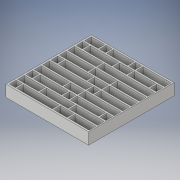
# Autodesk Inventor part: gitter
Saved by Autodesk Inventor 2017 (Build 210142000, 142)
## iProperties
Part Number: gitter
Material: Generisch
Document SubType Name: Modeling
Designer: Primaten
Density: 1 g/cm^3
Appearance: Vorgabe
Author: Primaten
Autodesk Inventor part; units mm, degrees
ref_plane "YZ Plane" through (0, 0, 0) normal (1, 0, 0) x (0, 1, 0)
ref_plane "XZ Plane" through (0, 0, 0) normal (0, 1, 0) x (-1, 0, 0)
ref_plane "XY Plane" through (0, 0, 0) normal (0, 0, 1) x (1, 0, 0)
sketch "Skizze1" plane through (0, 0, 0) normal (0, 0, 1) x (1, 0, 0)
  line L0 (-28.66, 0) -> (171.96, 0) construction
  line L1 (0, -29.6) -> (0, 177.6) construction
  line L2 (3, 3) -> (13.3, 3) construction
  line L3 (13.3, 3) -> (13.3, 14.5) construction
  line L4 (13.3, 14.5) -> (3, 14.5) construction
  line L5 (3, 14.5) -> (3, 3) construction
  line L6 (15.8, 3) -> (26.1, 3) construction
  line L7 (15.8, 14.5) -> (15.8, 3) construction
  line L8 (26.1, 14.5) -> (15.8, 14.5) construction
  line L9 (26.1, 3) -> (26.1, 14.5) construction
  line L10 (28.6, 3) -> (38.9, 3) construction
  line L11 (28.6, 14.5) -> (28.6, 3) construction
  line L12 (38.9, 14.5) -> (28.6, 14.5) construction
  line L13 (38.9, 3) -> (38.9, 14.5) construction
  line L14 (41.4, 3) -> (51.7, 3) construction
  line L15 (41.4, 14.5) -> (41.4, 3) construction
  line L16 (51.7, 14.5) -> (41.4, 14.5) construction
  line L17 (51.7, 3) -> (51.7, 14.5) construction
  line L18 (54.2, 3) -> (64.5, 3) construction
  line L19 (54.2, 14.5) -> (54.2, 3) construction
  line L20 (64.5, 14.5) -> (54.2, 14.5) construction
  line L21 (64.5, 3) -> (64.5, 14.5) construction
  line L22 (67, 3) -> (77.3, 3) construction
  line L23 (67, 14.5) -> (67, 3) construction
  line L24 (77.3, 14.5) -> (67, 14.5) construction
  line L25 (77.3, 3) -> (77.3, 14.5) construction
  line L26 (79.8, 3) -> (90.1, 3) construction
  line L27 (79.8, 14.5) -> (79.8, 3) construction
  line L28 (90.1, 14.5) -> (79.8, 14.5) construction
  line L29 (90.1, 3) -> (90.1, 14.5) construction
  line L30 (92.6, 3) -> (102.9, 3) construction
  line L31 (92.6, 14.5) -> (92.6, 3) construction
  line L32 (102.9, 14.5) -> (92.6, 14.5) construction
  line L33 (102.9, 3) -> (102.9, 14.5) construction
  line L34 (105.4, 3) -> (115.7, 3) construction
  line L35 (105.4, 14.5) -> (105.4, 3) construction
  line L36 (115.7, 14.5) -> (105.4, 14.5) construction
  line L37 (115.7, 3) -> (115.7, 14.5) construction
  line L38 (118.2, 3) -> (128.5, 3) construction
  line L39 (118.2, 14.5) -> (118.2, 3) construction
  line L40 (128.5, 14.5) -> (118.2, 14.5) construction
  line L41 (128.5, 3) -> (128.5, 14.5) construction
  line L42 (131, 3) -> (141.3, 3) construction
  line L43 (131, 14.5) -> (131, 3) construction
  line L44 (141.3, 14.5) -> (131, 14.5) construction
  line L45 (141.3, 3) -> (141.3, 14.5) construction
  line L46 (3, 17.5) -> (13.3, 17.5) construction
  line L47 (3, 29) -> (3, 17.5) construction
  line L48 (13.3, 29) -> (3, 29) construction
  line L49 (13.3, 17.5) -> (13.3, 29) construction
  line L50 (15.8, 17.5) -> (26.1, 17.5) construction
  line L51 (15.8, 29) -> (15.8, 17.5) construction
  line L52 (26.1, 29) -> (15.8, 29) construction
  line L53 (26.1, 17.5) -> (26.1, 29) construction
  line L54 (28.6, 17.5) -> (38.9, 17.5) construction
  line L55 (28.6, 29) -> (28.6, 17.5) construction
  line L56 (38.9, 29) -> (28.6, 29) construction
  line L57 (38.9, 17.5) -> (38.9, 29) construction
  line L58 (41.4, 17.5) -> (51.7, 17.5) construction
  line L59 (41.4, 29) -> (41.4, 17.5) construction
  line L60 (51.7, 29) -> (41.4, 29) construction
  line L61 (51.7, 17.5) -> (51.7, 29) construction
  line L62 (54.2, 17.5) -> (64.5, 17.5) construction
  line L63 (54.2, 29) -> (54.2, 17.5) construction
  line L64 (64.5, 29) -> (54.2, 29) construction
  line L65 (64.5, 17.5) -> (64.5, 29) construction
  line L66 (67, 17.5) -> (77.3, 17.5) construction
  line L67 (67, 29) -> (67, 17.5) construction
  line L68 (77.3, 29) -> (67, 29) construction
  line L69 (77.3, 17.5) -> (77.3, 29) construction
  line L70 (79.8, 17.5) -> (90.1, 17.5) construction
  line L71 (79.8, 29) -> (79.8, 17.5) construction
  line L72 (90.1, 29) -> (79.8, 29) construction
  line L73 (90.1, 17.5) -> (90.1, 29) construction
  line L74 (92.6, 17.5) -> (102.9, 17.5) construction
  line L75 (92.6, 29) -> (92.6, 17.5) construction
  line L76 (102.9, 29) -> (92.6, 29) construction
  line L77 (102.9, 17.5) -> (102.9, 29) construction
  line L78 (105.4, 17.5) -> (115.7, 17.5) construction
  line L79 (105.4, 29) -> (105.4, 17.5) construction
  line L80 (115.7, 29) -> (105.4, 29) construction
  line L81 (115.7, 17.5) -> (115.7, 29) construction
  line L82 (118.2, 17.5) -> (128.5, 17.5) construction
  line L83 (118.2, 29) -> (118.2, 17.5) construction
  line L84 (128.5, 29) -> (118.2, 29) construction
  line L85 (128.5, 17.5) -> (128.5, 29) construction
  line L86 (131, 17.5) -> (141.3, 17.5) construction
  line L87 (131, 29) -> (131, 17.5) construction
  line L88 (141.3, 29) -> (131, 29) construction
  line L89 (141.3, 17.5) -> (141.3, 29) construction
  line L90 (3, 32) -> (13.3, 32) construction
  line L91 (3, 43.5) -> (3, 32) construction
  line L92 (13.3, 43.5) -> (3, 43.5) construction
  line L93 (13.3, 32) -> (13.3, 43.5) construction
  line L94 (15.8, 32) -> (26.1, 32) construction
  line L95 (15.8, 43.5) -> (15.8, 32) construction
  line L96 (26.1, 43.5) -> (15.8, 43.5) construction
  line L97 (26.1, 32) -> (26.1, 43.5) construction
  line L98 (28.6, 32) -> (38.9, 32) construction
  line L99 (28.6, 43.5) -> (28.6, 32) construction
  line L100 (38.9, 43.5) -> (28.6, 43.5) construction
  line L101 (38.9, 32) -> (38.9, 43.5) construction
  line L102 (41.4, 32) -> (51.7, 32) construction
  line L103 (41.4, 43.5) -> (41.4, 32) construction
  line L104 (51.7, 43.5) -> (41.4, 43.5) construction
  line L105 (51.7, 32) -> (51.7, 43.5) construction
  line L106 (54.2, 32) -> (64.5, 32) construction
  line L107 (54.2, 43.5) -> (54.2, 32) construction
  line L108 (64.5, 43.5) -> (54.2, 43.5) construction
  line L109 (64.5, 32) -> (64.5, 43.5) construction
  line L110 (67, 32) -> (77.3, 32) construction
  line L111 (67, 43.5) -> (67, 32) construction
  line L112 (77.3, 43.5) -> (67, 43.5) construction
  line L113 (77.3, 32) -> (77.3, 43.5) construction
  line L114 (79.8, 32) -> (90.1, 32) construction
  line L115 (79.8, 43.5) -> (79.8, 32) construction
  line L116 (90.1, 43.5) -> (79.8, 43.5) construction
  line L117 (90.1, 32) -> (90.1, 43.5) construction
  line L118 (92.6, 32) -> (102.9, 32) construction
  line L119 (92.6, 43.5) -> (92.6, 32) construction
  line L120 (102.9, 43.5) -> (92.6, 43.5) construction
  line L121 (102.9, 32) -> (102.9, 43.5) construction
  line L122 (105.4, 32) -> (115.7, 32) construction
  line L123 (105.4, 43.5) -> (105.4, 32) construction
  line L124 (115.7, 43.5) -> (105.4, 43.5) construction
  line L125 (115.7, 32) -> (115.7, 43.5) construction
  line L126 (118.2, 32) -> (128.5, 32) construction
  line L127 (118.2, 43.5) -> (118.2, 32) construction
  line L128 (128.5, 43.5) -> (118.2, 43.5) construction
  line L129 (128.5, 32) -> (128.5, 43.5) construction
  line L130 (131, 32) -> (141.3, 32) construction
  line L131 (131, 43.5) -> (131, 32) construction
  line L132 (141.3, 43.5) -> (131, 43.5) construction
  line L133 (141.3, 32) -> (141.3, 43.5) construction
  line L134 (3, 46.5) -> (13.3, 46.5) construction
  line L135 (3, 58) -> (3, 46.5) construction
  line L136 (13.3, 58) -> (3, 58) construction
  line L137 (13.3, 46.5) -> (13.3, 58) construction
  line L138 (15.8, 46.5) -> (26.1, 46.5) construction
  line L139 (15.8, 58) -> (15.8, 46.5) construction
  line L140 (26.1, 58) -> (15.8, 58) construction
  line L141 (26.1, 46.5) -> (26.1, 58) construction
  line L142 (28.6, 46.5) -> (38.9, 46.5) construction
  line L143 (28.6, 58) -> (28.6, 46.5) construction
  line L144 (38.9, 58) -> (28.6, 58) construction
  line L145 (38.9, 46.5) -> (38.9, 58) construction
  line L146 (41.4, 46.5) -> (51.7, 46.5) construction
  line L147 (41.4, 58) -> (41.4, 46.5) construction
  line L148 (51.7, 58) -> (41.4, 58) construction
  line L149 (51.7, 46.5) -> (51.7, 58) construction
  line L150 (54.2, 46.5) -> (64.5, 46.5) construction
  line L151 (54.2, 58) -> (54.2, 46.5) construction
  line L152 (64.5, 58) -> (54.2, 58) construction
  line L153 (64.5, 46.5) -> (64.5, 58) construction
  line L154 (67, 46.5) -> (77.3, 46.5) construction
  line L155 (67, 58) -> (67, 46.5) construction
  line L156 (77.3, 58) -> (67, 58) construction
  line L157 (77.3, 46.5) -> (77.3, 58) construction
  line L158 (79.8, 46.5) -> (90.1, 46.5) construction
  line L159 (79.8, 58) -> (79.8, 46.5) construction
  line L160 (90.1, 58) -> (79.8, 58) construction
  line L161 (90.1, 46.5) -> (90.1, 58) construction
  line L162 (92.6, 46.5) -> (102.9, 46.5) construction
  line L163 (92.6, 58) -> (92.6, 46.5) construction
  line L164 (102.9, 58) -> (92.6, 58) construction
  line L165 (102.9, 46.5) -> (102.9, 58) construction
  line L166 (105.4, 46.5) -> (115.7, 46.5) construction
  line L167 (105.4, 58) -> (105.4, 46.5) construction
  line L168 (115.7, 58) -> (105.4, 58) construction
  line L169 (115.7, 46.5) -> (115.7, 58) construction
  line L170 (118.2, 46.5) -> (128.5, 46.5) construction
  line L171 (118.2, 58) -> (118.2, 46.5) construction
  line L172 (128.5, 58) -> (118.2, 58) construction
  line L173 (128.5, 46.5) -> (128.5, 58) construction
  line L174 (131, 46.5) -> (141.3, 46.5) construction
  line L175 (131, 58) -> (131, 46.5) construction
  line L176 (141.3, 58) -> (131, 58) construction
  line L177 (141.3, 46.5) -> (141.3, 58) construction
  line L178 (3, 61) -> (13.3, 61) construction
  line L179 (3, 72.5) -> (3, 61) construction
  line L180 (13.3, 72.5) -> (3, 72.5) construction
  line L181 (13.3, 61) -> (13.3, 72.5) construction
  line L182 (15.8, 61) -> (26.1, 61) construction
  line L183 (15.8, 72.5) -> (15.8, 61) construction
  line L184 (26.1, 72.5) -> (15.8, 72.5) construction
  line L185 (26.1, 61) -> (26.1, 72.5) construction
  line L186 (28.6, 61) -> (38.9, 61) construction
  line L187 (28.6, 72.5) -> (28.6, 61) construction
  line L188 (38.9, 72.5) -> (28.6, 72.5) construction
  line L189 (38.9, 61) -> (38.9, 72.5) construction
  line L190 (41.4, 61) -> (51.7, 61) construction
  line L191 (41.4, 72.5) -> (41.4, 61) construction
  line L192 (51.7, 72.5) -> (41.4, 72.5) construction
  line L193 (51.7, 61) -> (51.7, 72.5) construction
  line L194 (54.2, 61) -> (64.5, 61) construction
  line L195 (54.2, 72.5) -> (54.2, 61) construction
  line L196 (64.5, 72.5) -> (54.2, 72.5) construction
  line L197 (64.5, 61) -> (64.5, 72.5) construction
  line L198 (67, 61) -> (77.3, 61) construction
  line L199 (67, 72.5) -> (67, 61) construction
  line L200 (77.3, 72.5) -> (67, 72.5) construction
  line L201 (77.3, 61) -> (77.3, 72.5) construction
  line L202 (79.8, 61) -> (90.1, 61) construction
  line L203 (79.8, 72.5) -> (79.8, 61) construction
  line L204 (90.1, 72.5) -> (79.8, 72.5) construction
  line L205 (90.1, 61) -> (90.1, 72.5) construction
  line L206 (92.6, 61) -> (102.9, 61) construction
  line L207 (92.6, 72.5) -> (92.6, 61) construction
  line L208 (102.9, 72.5) -> (92.6, 72.5) construction
  line L209 (102.9, 61) -> (102.9, 72.5) construction
  line L210 (105.4, 61) -> (115.7, 61) construction
  line L211 (105.4, 72.5) -> (105.4, 61) construction
  line L212 (115.7, 72.5) -> (105.4, 72.5) construction
  line L213 (115.7, 61) -> (115.7, 72.5) construction
  line L214 (118.2, 61) -> (128.5, 61) construction
  line L215 (118.2, 72.5) -> (118.2, 61) construction
  line L216 (128.5, 72.5) -> (118.2, 72.5) construction
  line L217 (128.5, 61) -> (128.5, 72.5) construction
  line L218 (131, 61) -> (141.3, 61) construction
  line L219 (131, 72.5) -> (131, 61) construction
  line L220 (141.3, 72.5) -> (131, 72.5) construction
  line L221 (141.3, 61) -> (141.3, 72.5) construction
  line L222 (3, 75.5) -> (13.3, 75.5) construction
  line L223 (3, 87) -> (3, 75.5) construction
  line L224 (13.3, 87) -> (3, 87) construction
  line L225 (13.3, 75.5) -> (13.3, 87) construction
  line L226 (15.8, 75.5) -> (26.1, 75.5) construction
  line L227 (15.8, 87) -> (15.8, 75.5) construction
  line L228 (26.1, 87) -> (15.8, 87) construction
  line L229 (26.1, 75.5) -> (26.1, 87) construction
  line L230 (28.6, 75.5) -> (38.9, 75.5) construction
  line L231 (28.6, 87) -> (28.6, 75.5) construction
  line L232 (38.9, 87) -> (28.6, 87) construction
  line L233 (38.9, 75.5) -> (38.9, 87) construction
  line L234 (41.4, 75.5) -> (51.7, 75.5) construction
  line L235 (41.4, 87) -> (41.4, 75.5) construction
  line L236 (51.7, 87) -> (41.4, 87) construction
  line L237 (51.7, 75.5) -> (51.7, 87) construction
  line L238 (54.2, 75.5) -> (64.5, 75.5) construction
  line L239 (54.2, 87) -> (54.2, 75.5) construction
  line L240 (64.5, 87) -> (54.2, 87) construction
  line L241 (64.5, 75.5) -> (64.5, 87) construction
  line L242 (67, 75.5) -> (77.3, 75.5) construction
  line L243 (67, 87) -> (67, 75.5) construction
  line L244 (77.3, 87) -> (67, 87) construction
  line L245 (77.3, 75.5) -> (77.3, 87) construction
  line L246 (79.8, 75.5) -> (90.1, 75.5) construction
  line L247 (79.8, 87) -> (79.8, 75.5) construction
  line L248 (90.1, 87) -> (79.8, 87) construction
  line L249 (90.1, 75.5) -> (90.1, 87) construction
  line L250 (92.6, 75.5) -> (102.9, 75.5) construction
  line L251 (92.6, 87) -> (92.6, 75.5) construction
  line L252 (102.9, 87) -> (92.6, 87) construction
  line L253 (102.9, 75.5) -> (102.9, 87) construction
  line L254 (105.4, 75.5) -> (115.7, 75.5) construction
  line L255 (105.4, 87) -> (105.4, 75.5) construction
  line L256 (115.7, 87) -> (105.4, 87) construction
  line L257 (115.7, 75.5) -> (115.7, 87) construction
  line L258 (118.2, 75.5) -> (128.5, 75.5) construction
  line L259 (118.2, 87) -> (118.2, 75.5) construction
  line L260 (128.5, 87) -> (118.2, 87) construction
  line L261 (128.5, 75.5) -> (128.5, 87) construction
  line L262 (131, 75.5) -> (141.3, 75.5) construction
  line L263 (131, 87) -> (131, 75.5) construction
  line L264 (141.3, 87) -> (131, 87) construction
  line L265 (141.3, 75.5) -> (141.3, 87) construction
  line L266 (3, 90) -> (13.3, 90) construction
  line L267 (3, 101.5) -> (3, 90) construction
  line L268 (13.3, 101.5) -> (3, 101.5) construction
  line L269 (13.3, 90) -> (13.3, 101.5) construction
  line L270 (15.8, 90) -> (26.1, 90) construction
  line L271 (15.8, 101.5) -> (15.8, 90) construction
  line L272 (26.1, 101.5) -> (15.8, 101.5) construction
  line L273 (26.1, 90) -> (26.1, 101.5) construction
  line L274 (28.6, 90) -> (38.9, 90) construction
  line L275 (28.6, 101.5) -> (28.6, 90) construction
  line L276 (38.9, 101.5) -> (28.6, 101.5) construction
  line L277 (38.9, 90) -> (38.9, 101.5) construction
  line L278 (41.4, 90) -> (51.7, 90) construction
  line L279 (41.4, 101.5) -> (41.4, 90) construction
  line L280 (51.7, 101.5) -> (41.4, 101.5) construction
  line L281 (51.7, 90) -> (51.7, 101.5) construction
  line L282 (54.2, 90) -> (64.5, 90) construction
  line L283 (54.2, 101.5) -> (54.2, 90) construction
  line L284 (64.5, 101.5) -> (54.2, 101.5) construction
  line L285 (64.5, 90) -> (64.5, 101.5) construction
  line L286 (67, 90) -> (77.3, 90) construction
  line L287 (67, 101.5) -> (67, 90) construction
  line L288 (77.3, 101.5) -> (67, 101.5) construction
  line L289 (77.3, 90) -> (77.3, 101.5) construction
  line L290 (79.8, 90) -> (90.1, 90) construction
  line L291 (79.8, 101.5) -> (79.8, 90) construction
  line L292 (90.1, 101.5) -> (79.8, 101.5) construction
  line L293 (90.1, 90) -> (90.1, 101.5) construction
  line L294 (92.6, 90) -> (102.9, 90) construction
  line L295 (92.6, 101.5) -> (92.6, 90) construction
  line L296 (102.9, 101.5) -> (92.6, 101.5) construction
  line L297 (102.9, 90) -> (102.9, 101.5) construction
  line L298 (105.4, 90) -> (115.7, 90) construction
  line L299 (105.4, 101.5) -> (105.4, 90) construction
  line L300 (115.7, 101.5) -> (105.4, 101.5) construction
  line L301 (115.7, 90) -> (115.7, 101.5) construction
  line L302 (118.2, 90) -> (128.5, 90) construction
  line L303 (118.2, 101.5) -> (118.2, 90) construction
  line L304 (128.5, 101.5) -> (118.2, 101.5) construction
  line L305 (128.5, 90) -> (128.5, 101.5) construction
  line L306 (131, 90) -> (141.3, 90) construction
  line L307 (131, 101.5) -> (131, 90) construction
  line L308 (141.3, 101.5) -> (131, 101.5) construction
  line L309 (141.3, 90) -> (141.3, 101.5) construction
  line L310 (3, 104.5) -> (13.3, 104.5) construction
  line L311 (3, 116) -> (3, 104.5) construction
  line L312 (13.3, 116) -> (3, 116) construction
  line L313 (13.3, 104.5) -> (13.3, 116) construction
  line L314 (15.8, 104.5) -> (26.1, 104.5) construction
  line L315 (15.8, 116) -> (15.8, 104.5) construction
  line L316 (26.1, 116) -> (15.8, 116) construction
  line L317 (26.1, 104.5) -> (26.1, 116) construction
  line L318 (28.6, 104.5) -> (38.9, 104.5) construction
  line L319 (28.6, 116) -> (28.6, 104.5) construction
  line L320 (38.9, 116) -> (28.6, 116) construction
  line L321 (38.9, 104.5) -> (38.9, 116) construction
  line L322 (41.4, 104.5) -> (51.7, 104.5) construction
  line L323 (41.4, 116) -> (41.4, 104.5) construction
  line L324 (51.7, 116) -> (41.4, 116) construction
  line L325 (51.7, 104.5) -> (51.7, 116) construction
  line L326 (54.2, 104.5) -> (64.5, 104.5) construction
  line L327 (54.2, 116) -> (54.2, 104.5) construction
  line L328 (64.5, 116) -> (54.2, 116) construction
  line L329 (64.5, 104.5) -> (64.5, 116) construction
  line L330 (67, 104.5) -> (77.3, 104.5) construction
  line L331 (67, 116) -> (67, 104.5) construction
  line L332 (77.3, 116) -> (67, 116) construction
  line L333 (77.3, 104.5) -> (77.3, 116) construction
  line L334 (79.8, 104.5) -> (90.1, 104.5) construction
  line L335 (79.8, 116) -> (79.8, 104.5) construction
  line L336 (90.1, 116) -> (79.8, 116) construction
  line L337 (90.1, 104.5) -> (90.1, 116) construction
  line L338 (92.6, 104.5) -> (102.9, 104.5) construction
  line L339 (92.6, 116) -> (92.6, 104.5) construction
  line L340 (102.9, 116) -> (92.6, 116) construction
  line L341 (102.9, 104.5) -> (102.9, 116) construction
  line L342 (105.4, 104.5) -> (115.7, 104.5) construction
  line L343 (105.4, 116) -> (105.4, 104.5) construction
  line L344 (115.7, 116) -> (105.4, 116) construction
  line L345 (115.7, 104.5) -> (115.7, 116) construction
  line L346 (118.2, 104.5) -> (128.5, 104.5) construction
  line L347 (118.2, 116) -> (118.2, 104.5) construction
  line L348 (128.5, 116) -> (118.2, 116) construction
  line L349 (128.5, 104.5) -> (128.5, 116) construction
  line L350 (131, 104.5) -> (141.3, 104.5) construction
  line L351 (131, 116) -> (131, 104.5) construction
  line L352 (141.3, 116) -> (131, 116) construction
  line L353 (141.3, 104.5) -> (141.3, 116) construction
  line L354 (3, 119) -> (13.3, 119) construction
  line L355 (3, 130.5) -> (3, 119) construction
  line L356 (13.3, 130.5) -> (3, 130.5) construction
  line L357 (13.3, 119) -> (13.3, 130.5) construction
  line L358 (15.8, 119) -> (26.1, 119) construction
  line L359 (15.8, 130.5) -> (15.8, 119) construction
  line L360 (26.1, 130.5) -> (15.8, 130.5) construction
  line L361 (26.1, 119) -> (26.1, 130.5) construction
  line L362 (28.6, 119) -> (38.9, 119) construction
  line L363 (28.6, 130.5) -> (28.6, 119) construction
  line L364 (38.9, 130.5) -> (28.6, 130.5) construction
  line L365 (38.9, 119) -> (38.9, 130.5) construction
  line L366 (41.4, 119) -> (51.7, 119) construction
  line L367 (41.4, 130.5) -> (41.4, 119) construction
  line L368 (51.7, 130.5) -> (41.4, 130.5) construction
  line L369 (51.7, 119) -> (51.7, 130.5) construction
  line L370 (54.2, 119) -> (64.5, 119) construction
  line L371 (54.2, 130.5) -> (54.2, 119) construction
  line L372 (64.5, 130.5) -> (54.2, 130.5) construction
  line L373 (64.5, 119) -> (64.5, 130.5) construction
  line L374 (67, 119) -> (77.3, 119) construction
  line L375 (67, 130.5) -> (67, 119) construction
  line L376 (77.3, 130.5) -> (67, 130.5) construction
  line L377 (77.3, 119) -> (77.3, 130.5) construction
  line L378 (79.8, 119) -> (90.1, 119) construction
  line L379 (79.8, 130.5) -> (79.8, 119) construction
  line L380 (90.1, 130.5) -> (79.8, 130.5) construction
  line L381 (90.1, 119) -> (90.1, 130.5) construction
  line L382 (92.6, 119) -> (102.9, 119) construction
  line L383 (92.6, 130.5) -> (92.6, 119) construction
  line L384 (102.9, 130.5) -> (92.6, 130.5) construction
  line L385 (102.9, 119) -> (102.9, 130.5) construction
  line L386 (105.4, 119) -> (115.7, 119) construction
  line L387 (105.4, 130.5) -> (105.4, 119) construction
  line L388 (115.7, 130.5) -> (105.4, 130.5) construction
  line L389 (115.7, 119) -> (115.7, 130.5) construction
  line L390 (118.2, 119) -> (128.5, 119) construction
  line L391 (118.2, 130.5) -> (118.2, 119) construction
  line L392 (128.5, 130.5) -> (118.2, 130.5) construction
  line L393 (128.5, 119) -> (128.5, 130.5) construction
  line L394 (131, 119) -> (141.3, 119) construction
  line L395 (131, 130.5) -> (131, 119) construction
  line L396 (141.3, 130.5) -> (131, 130.5) construction
  line L397 (141.3, 119) -> (141.3, 130.5) construction
  line L398 (3, 133.5) -> (13.3, 133.5) construction
  line L399 (3, 145) -> (3, 133.5) construction
  line L400 (13.3, 145) -> (3, 145) construction
  line L401 (13.3, 133.5) -> (13.3, 145) construction
  line L402 (15.8, 133.5) -> (26.1, 133.5) construction
  line L403 (15.8, 145) -> (15.8, 133.5) construction
  line L404 (26.1, 145) -> (15.8, 145) construction
  line L405 (26.1, 133.5) -> (26.1, 145) construction
  line L406 (28.6, 133.5) -> (38.9, 133.5) construction
  line L407 (28.6, 145) -> (28.6, 133.5) construction
  line L408 (38.9, 145) -> (28.6, 145) construction
  line L409 (38.9, 133.5) -> (38.9, 145) construction
  line L410 (41.4, 133.5) -> (51.7, 133.5) construction
  line L411 (41.4, 145) -> (41.4, 133.5) construction
  line L412 (51.7, 145) -> (41.4, 145) construction
  line L413 (51.7, 133.5) -> (51.7, 145) construction
  line L414 (54.2, 133.5) -> (64.5, 133.5) construction
  line L415 (54.2, 145) -> (54.2, 133.5) construction
  line L416 (64.5, 145) -> (54.2, 145) construction
  line L417 (64.5, 133.5) -> (64.5, 145) construction
  line L418 (67, 133.5) -> (77.3, 133.5) construction
  line L419 (67, 145) -> (67, 133.5) construction
  line L420 (77.3, 145) -> (67, 145) construction
  line L421 (77.3, 133.5) -> (77.3, 145) construction
  line L422 (79.8, 133.5) -> (90.1, 133.5) construction
  line L423 (79.8, 145) -> (79.8, 133.5) construction
  line L424 (90.1, 145) -> (79.8, 145) construction
  line L425 (90.1, 133.5) -> (90.1, 145) construction
  line L426 (92.6, 133.5) -> (102.9, 133.5) construction
  line L427 (92.6, 145) -> (92.6, 133.5) construction
  line L428 (102.9, 145) -> (92.6, 145) construction
  line L429 (102.9, 133.5) -> (102.9, 145) construction
  line L430 (105.4, 133.5) -> (115.7, 133.5) construction
  line L431 (105.4, 145) -> (105.4, 133.5) construction
  line L432 (115.7, 145) -> (105.4, 145) construction
  line L433 (115.7, 133.5) -> (115.7, 145) construction
  line L434 (118.2, 133.5) -> (128.5, 133.5) construction
  line L435 (118.2, 145) -> (118.2, 133.5) construction
  line L436 (128.5, 145) -> (118.2, 145) construction
  line L437 (128.5, 133.5) -> (128.5, 145) construction
  line L438 (131, 133.5) -> (141.3, 133.5) construction
  line L439 (131, 145) -> (131, 133.5) construction
  line L440 (141.3, 145) -> (131, 145) construction
  line L441 (141.3, 133.5) -> (141.3, 145) construction
  line L442 (0, 0) -> (143.3, 0) construction
  line L443 (143.3, 0) -> (143.3, 148) construction
  line L444 (143.3, 148) -> (0, 148) construction
  line L445 (0, 148) -> (0, 0) construction
  line L446 (0, 0) -> (143.3, 0)
  line L447 (143.3, 0) -> (143.3, 148)
  line L448 (143.3, 148) -> (0, 148)
  line L449 (0, 148) -> (0, 0)
  line L450 (3, 145) -> (26.1, 145)
  line L451 (26.1, 145) -> (26.1, 133.5)
  line L452 (26.1, 133.5) -> (3, 133.5)
  line L453 (3, 133.5) -> (3, 145)
  line L454 (28.6, 145) -> (38.9, 145)
  line L455 (38.9, 145) -> (38.9, 133.5)
  line L456 (38.9, 133.5) -> (28.6, 133.5)
  line L457 (28.6, 133.5) -> (28.6, 145)
  line L458 (41.4, 145) -> (77.3, 145)
  line L459 (77.3, 145) -> (77.3, 133.5)
  line L460 (77.3, 133.5) -> (41.4, 133.5)
  line L461 (41.4, 133.5) -> (41.4, 145)
  line L462 (79.8, 145) -> (90.1, 145)
  line L463 (90.1, 145) -> (90.1, 133.5)
  line L464 (90.1, 133.5) -> (79.8, 133.5)
  line L465 (79.8, 133.5) -> (79.8, 145)
  line L466 (90.1, 130.5) -> (67, 130.5)
  line L467 (67, 130.5) -> (67, 119)
  line L468 (67, 119) -> (90.1, 119)
  line L469 (90.1, 119) -> (90.1, 130.5)
  line L470 (92.6, 133.5) -> (141.3, 133.5)
  line L471 (141.3, 133.5) -> (141.3, 145)
  line L472 (141.3, 145) -> (92.6, 145)
  line L473 (92.6, 145) -> (92.6, 133.5)
  line L474 (131, 130.5) -> (141.3, 130.5)
  line L475 (141.3, 130.5) -> (141.3, 119)
  line L476 (141.3, 119) -> (131, 119)
  line L477 (131, 119) -> (131, 130.5)
  line L478 (128.5, 130.5) -> (92.6, 130.5)
  line L479 (92.6, 130.5) -> (92.6, 119)
  line L480 (92.6, 119) -> (128.5, 119)
  line L481 (128.5, 119) -> (128.5, 130.5)
  line L482 (51.7, 116) -> (3, 116)
  line L483 (3, 116) -> (3, 104.5)
  line L484 (3, 104.5) -> (51.7, 104.5)
  line L485 (51.7, 104.5) -> (51.7, 116)
  line L486 (54.2, 116) -> (141.3, 116)
  line L487 (141.3, 116) -> (141.3, 104.5)
  line L488 (141.3, 104.5) -> (54.2, 104.5)
  line L489 (54.2, 104.5) -> (54.2, 116)
  line L490 (13.3, 130.5) -> (3, 130.5)
  line L491 (3, 130.5) -> (3, 119)
  line L492 (3, 119) -> (13.3, 119)
  line L493 (13.3, 119) -> (13.3, 130.5)
  line L494 (15.8, 119) -> (64.5, 119)
  line L495 (64.5, 119) -> (64.5, 130.5)
  line L496 (64.5, 130.5) -> (15.8, 130.5)
  line L497 (15.8, 130.5) -> (15.8, 119)
  line L498 (51.7, 101.5) -> (3, 101.5)
  line L499 (3, 101.5) -> (3, 90)
  line L500 (3, 90) -> (51.7, 90)
  line L501 (51.7, 90) -> (51.7, 101.5)
  line L502 (54.2, 101.5) -> (90.1, 101.5)
  line L503 (90.1, 101.5) -> (90.1, 90)
  line L504 (90.1, 90) -> (54.2, 90)
  line L505 (54.2, 90) -> (54.2, 101.5)
  line L506 (92.6, 101.5) -> (141.3, 101.5)
  line L507 (141.3, 101.5) -> (141.3, 90)
  line L508 (141.3, 90) -> (92.6, 90)
  line L509 (92.6, 90) -> (92.6, 101.5)
  line L510 (3, 87) -> (13.3, 87)
  line L511 (13.3, 87) -> (13.3, 75.5)
  line L512 (13.3, 75.5) -> (3, 75.5)
  line L513 (3, 75.5) -> (3, 87)
  line L514 (15.8, 87) -> (64.5, 87)
  line L515 (64.5, 87) -> (64.5, 75.5)
  line L516 (64.5, 75.5) -> (15.8, 75.5)
  line L517 (15.8, 75.5) -> (15.8, 87)
  line L518 (67, 87) -> (90.1, 87)
  line L519 (90.1, 87) -> (90.1, 75.5)
  line L520 (90.1, 75.5) -> (67, 75.5)
  line L521 (67, 75.5) -> (67, 87)
  line L522 (92.6, 87) -> (141.3, 87)
  line L523 (141.3, 87) -> (141.3, 75.5)
  line L524 (141.3, 75.5) -> (92.6, 75.5)
  line L525 (92.6, 75.5) -> (92.6, 87)
  line L526 (79.8, 72.5) -> (90.1, 72.5)
  line L527 (90.1, 72.5) -> (90.1, 61)
  line L528 (90.1, 61) -> (79.8, 61)
  line L529 (79.8, 61) -> (79.8, 72.5)
  line L530 (92.6, 61) -> (141.3, 61)
  line L531 (141.3, 61) -> (141.3, 72.5)
  line L532 (141.3, 72.5) -> (92.6, 72.5)
  line L533 (92.6, 72.5) -> (92.6, 61)
  line L534 (77.3, 72.5) -> (3, 72.5)
  line L535 (3, 72.5) -> (3, 61)
  line L536 (3, 61) -> (77.3, 61)
  line L537 (77.3, 61) -> (77.3, 72.5)
  line L538 (3, 58) -> (51.7, 58)
  line L539 (51.7, 58) -> (51.7, 46.5)
  line L540 (51.7, 46.5) -> (3, 46.5)
  line L541 (3, 46.5) -> (3, 58)
  line L542 (54.2, 58) -> (77.3, 58)
  line L543 (77.3, 58) -> (77.3, 46.5)
  line L544 (77.3, 46.5) -> (54.2, 46.5)
  line L545 (54.2, 46.5) -> (54.2, 58)
  line L546 (79.8, 58) -> (141.3, 58)
  line L547 (141.3, 58) -> (141.3, 46.5)
  line L548 (141.3, 46.5) -> (79.8, 46.5)
  line L549 (79.8, 46.5) -> (79.8, 58)
  line L550 (77.3, 43.5) -> (67, 43.5)
  line L551 (67, 43.5) -> (67, 32)
  line L552 (67, 32) -> (77.3, 32)
  line L553 (77.3, 32) -> (77.3, 43.5)
  line L554 (64.5, 43.5) -> (15.8, 43.5)
  line L555 (15.8, 43.5) -> (15.8, 32)
  line L556 (15.8, 32) -> (64.5, 32)
  line L557 (64.5, 32) -> (64.5, 43.5)
  line L558 (13.3, 43.5) -> (3, 43.5)
  line L559 (3, 43.5) -> (3, 32)
  line L560 (3, 32) -> (13.3, 32)
  line L561 (13.3, 32) -> (13.3, 43.5)
  line L562 (79.8, 43.5) -> (128.5, 43.5)
  line L563 (141.3, 43.5) -> (141.3, 32)
  line L564 (141.3, 32) -> (131, 32)
  line L565 (79.8, 32) -> (79.8, 43.5)
  line L566 (3, 29) -> (38.9, 29)
  line L567 (38.9, 29) -> (38.9, 17.5)
  line L568 (38.9, 17.5) -> (3, 17.5)
  line L569 (3, 17.5) -> (3, 29)
  line L570 (41.4, 29) -> (90.1, 29)
  line L571 (90.1, 29) -> (90.1, 17.5)
  line L572 (90.1, 17.5) -> (41.4, 17.5)
  line L573 (41.4, 17.5) -> (41.4, 29)
  line L574 (92.6, 29) -> (141.3, 29)
  line L575 (141.3, 29) -> (141.3, 17.5)
  line L576 (141.3, 17.5) -> (92.6, 17.5)
  line L577 (92.6, 17.5) -> (92.6, 29)
  line L578 (105.4, 14.5) -> (141.3, 14.5)
  line L579 (141.3, 14.5) -> (141.3, 3)
  line L580 (141.3, 3) -> (105.4, 3)
  line L581 (105.4, 3) -> (105.4, 14.5)
  line L582 (102.9, 14.5) -> (79.8, 14.5)
  line L583 (79.8, 14.5) -> (79.8, 3)
  line L584 (79.8, 3) -> (102.9, 3)
  line L585 (102.9, 3) -> (102.9, 14.5)
  line L586 (77.3, 14.5) -> (15.8, 14.5)
  line L587 (15.8, 14.5) -> (15.8, 3)
  line L588 (15.8, 3) -> (77.3, 3)
  line L589 (77.3, 3) -> (77.3, 14.5)
  line L590 (13.3, 3) -> (3, 3)
  line L591 (3, 3) -> (3, 14.5)
  line L592 (3, 14.5) -> (13.3, 14.5)
  line L593 (13.3, 14.5) -> (13.3, 3)
  line L594 (128.5, 32) -> (128.5, 43.5)
  line L595 (131, 43.5) -> (131, 32)
  line L596 (131, 43.5) -> (141.3, 43.5)
  line L597 (128.5, 32) -> (79.8, 32)
  dimension "a1" = 10.3
  dimension "b2" = 11.5
  dimension "c3" = 3
  dimension "d9" = 3
  dimension "d12" = 12.8
  dimension "d15" = 14.5
  dimension "hj" = 143.3
  dimension "hk" = 148
  constraints: 1192 end point, 81 parallel, 41 horizontal, 40 perpendicular, 3 vertical, 872 other
  measures "a1" distance of L4.end L3.end
  measures "b2" distance of L3.end L2.end
  measures "c3" distance from line of L0 L2.start
  measures "d9" distance from line of L1 L2.start
  measures "d12" distance of L2.start L6.start
  measures "d15" distance of L2.start L46.start
  measures "hj" distance of L444.end L443.end
  measures "hk" distance of L442.end L443.end
extrude "Extrusion3" add sketch "Skizze1" along normal blind 20
equation "\"c3\" = m4"
equation "\"d9\" = c3"
equation "\"d12\" = a1 + m3"
equation "\"d15\" = b2 + m4"
equation "\"hj\" = 11 * a1 + 12 * m3"
equation "\"hk\" = 10 * b2 + 11 * m4"
equation "\"m4\" = 3"
equation "\"m3\" = 2.5"
